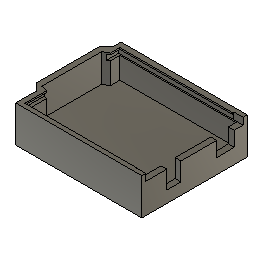
socle arduino Nathan_Dumand (Autodesk Fusion 360 design; units mm, degrees)
Autodesk Fusion 360 part; units mm, degrees
sketch "Esquisse1" plane through (0, 0, 0) normal (0, 0, 1) x (1, 0, 0) in component "socle"
  line L0 (-30.3825, 11.4148) -> (45.6175, 11.4148)
  line L1 (45.6175, 11.4148) -> (45.6175, 74.9148)
  line L2 (45.6175, 74.9148) -> (-30.3825, 74.9148)
  line L3 (-30.3825, 74.9148) -> (-30.3825, 70.0148)
  line L4 (-30.3825, 11.4148) -> (-30.3825, 23.9148)
  line L5 (-30.3825, 23.9148) -> (-34.567, 28.2148)
  line L6 (-34.567, 65.7148) -> (-30.3825, 70.0148)
  line L7 (-34.567, 65.7148) -> (-34.567, 28.2148)
  dimension "d1" = 76
  dimension "d2" = 63.5
  dimension "d3" = 4.9
  dimension "d4" = 12.5
  dimension "d5" = 37.5
  dimension "d19" = 6
  constraint horizontal L0
  constraint perpendicular L0 L1
  constraint perpendicular L1 L2
  constraint vertical L3
  constraint perpendicular L0 L4
  constraint equal L5 L6
  constraint equal L0 L2
  constraint vertical L7
  measures "d1" distance of L0.start L0.end
  measures "d2" distance of L0.end L1.end
  measures "d3" distance of L2.end L3.end
  measures "d4" distance of L0.start L4.end
  measures "d5" distance of L5.end L6.start
  measures "d19" distance of L3.end L6.start
extrude "Extrusion1" add sketch "Esquisse1" along normal blind 22 in component "socle"
sketch "Esquisse4" plane through (0, 0, 22) normal (0, 0, 1) x (-1, 0, 0) in component "socle"
  line L0 (30.3825, -11.4148) -> (-45.6175, -11.4148)
  line L1 (-45.6175, -11.4148) -> (-45.6175, -74.9148)
  line L2 (-45.6175, -74.9148) -> (30.3825, -74.9148)
  line L3 (30.3825, -74.9148) -> (30.3825, -70.0148)
  line L4 (30.3825, -70.0148) -> (34.567, -65.7148)
  line L5 (34.567, -28.2148) -> (30.3825, -23.9148)
  line L6 (30.3825, -23.9148) -> (30.3825, -11.4148)
  line L7 (-42.1196, -14) -> (-42.1196, -71.6421)
  line L8 (27.4232, -14) -> (27.4232, -27.0414)
  line L9 (27.8622, -71.6421) -> (27.8622, -66.0114)
  line L10 (31.2452, -63.9938) -> (31.2452, -27.9938)
  line L11 (31.2452, -63.9938) -> (27.8622, -66.0114)
  line L12 (31.2452, -27.9938) -> (27.4232, -27.0414)
  line L13 (27.4232, -14) -> (-42.1196, -14)
  line L14 (-42.1196, -71.6421) -> (27.8622, -71.6421)
  line L15 (34.567, -65.7148) -> (34.567, -28.2148)
  dimension "d9" = 3
  dimension "d13" = 36
  constraint vertical L10
  constraint equal L11 L12
  constraint parallel L1 L7
  constraint perpendicular L7 L13
  constraint perpendicular L9 L14
  constraint perpendicular L8 L13
  constraint perpendicular L7 L14
  measures "d9" distance of L3.end L9.start
  measures "d13" distance of L10.start L10.end
extrude "Extrusion2" cut sketch "Esquisse4" against normal blind 17 contours L7 L8 L9 L10 L11 L12 L13 L14 in component "socle"
sketch "Esquisse6" plane through (45.6175, 0, 0) normal (1, 0, 0) x (0, 1, 0) in component "socle"
  line L0 (74.9148, 22) -> (11.4148, 22)
  line L1 (11.4148, 22) -> (11.4148, 0)
  line L2 (11.4148, 0) -> (74.9148, 0)
  line L3 (74.9148, 0) -> (74.9148, 22)
  line L4 (13.8459, 17.9261) -> (13.8459, 21.0761)
  line L5 (13.8459, 17.9261) -> (72.4148, 17.9261)
  line L6 (72.4148, 17.9261) -> (72.4148, 21.0761)
  line L7 (72.4148, 21.0761) -> (13.8459, 21.0761)
  dimension "d33" = 3.15
  constraint perpendicular L5 L6
  constraint parallel L4 L6
  constraint parallel L5 L7
  measures "d33" distance of L4.start L4.end
extrude "Extrusion4" cut sketch "Esquisse6" against normal blind 75 contours L4 L5 L6 L7 in component "socle"
sketch "Esquisse5" plane through (45.6175, 0, 0) normal (1, 0, 0) x (0, 1, 0) in component "socle"
  line L0 (11.4148, 0) -> (74.9148, 0)
  line L1 (74.9148, 0) -> (74.9148, 22)
  line L2 (74.9148, 22) -> (11.4148, 22)
  line L3 (11.4148, 22) -> (11.4148, 0)
  line L4 (67.0675, 22) -> (56.569, 21.8233)
  line L5 (34.9761, 7) -> (26.4761, 7)
  line L6 (56.5452, 8.8233) -> (67.0411, 9.1144)
  line L7 (72.4148, 21.0761) -> (72.4148, 17.9261)
  line L8 (13.8459, 17.9261) -> (13.8459, 21.0761)
  line L9 (26.4761, 7) -> (26.4762, 17.9261)
  line L10 (34.9761, 7) -> (34.9776, 18.4994)
  line L11 (26.4762, 17.9261) -> (13.8459, 17.9261)
  line L12 (72.4148, 17.9261) -> (67.046, 17.9291)
  line L13 (56.5464, 18.4968) -> (34.9776, 18.4994)
  line L14 (13.8459, 17.9261) -> (13.8459, 22)
  line L15 (72.4171, 22) -> (72.4148, 17.9261)
  line L16 (72.4171, 22) -> (13.8459, 22)
  line L17 (56.5452, 8.8233) -> (56.5464, 18.4968)
  line L18 (67.0411, 9.1144) -> (67.046, 17.9291)
  dimension "d21" = 10.5
  dimension "d22" = 13
  dimension "d23" = 10.5
  dimension "d26" = 8.5
  constraint coincident L2 L4.start
  constraint coincident L8.start L11.end
  constraint perpendicular L8 L11
  constraint coincident L7.end L12.start
  constraint perpendicular L10 L13
  constraint coincident L2 L14.end
  constraint perpendicular L2 L14
  constraint coincident L2 L15.start
  constraint perpendicular L12 L15
  constraint perpendicular L13 L17
  constraint perpendicular L12 L18
  measures "d21" distance of L4.start L4.end
  measures "d22" distance of L4.end L6.start
  measures "d23" distance of L6.start L6.end
  measures "d26" distance of L5.start L5.end
extrude "Extrusion3" cut sketch "Esquisse5" against normal blind 5.5 contours L2 L5 L6 L7 L8 L9 L10 L11 L12 L13 L14 L15 L16 L17 L18 in component "socle"
component "socle" placed x (1, 0, 0) y (0, 1, 0) z (0, 0, 1) at (0, 0, 0)
equation "d6 = h"
equation "d33 = epv"
equation "h = 22 mm"
equation "epv = 3.15 mm"
